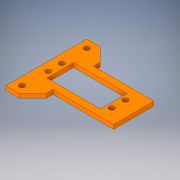
# Autodesk Inventor part: Pinza_sostenedor
Saved by Autodesk Inventor 2019 (Build 230136000, 136)
## iProperties
Created: 2020-02-07
Part Number: Pinza_sostenedor
Material: Generic
Document SubType Name: Modeling
Designer: Omar
Density: 1 g/cm^3
Appearance: Default
Author: Omar
Autodesk Inventor part; units mm, degrees
ref_plane "YZ Plane" through (0, 0, 0) normal (1, 0, 0) x (0, 1, 0)
ref_plane "XZ Plane" through (0, 0, 0) normal (0, 1, 0) x (-1, 0, 0)
ref_plane "XY Plane" through (0, 0, 0) normal (0, 0, 1) x (1, 0, 0)
sketch "Sketch2" plane through (0, 0, 0) normal (0, 1, 0) x (-1, 0, 0)
  circle A0 centre (-33.79, -5.085) radius 2
  circle A1 centre (-33.79, 5.085) radius 2
  circle A2 centre (13.47, -5.085) radius 2
  circle A3 centre (13.47, 5.085) radius 2
  line L0 (20, 15) -> (-45, 15)
  line L1 (-45, 15) -> (-45, -15)
  line L2 (-45, -15) -> (20, -15)
  line L3 (20, -15) -> (20, 15)
  line L4 (20, 30) -> (0, 30)
  line L5 (0, -30) -> (20, -30)
  line L6 (20, -30) -> (20, 30)
  circle A4 centre (14, 24) radius 2
  circle A5 centre (14, -24) radius 2
  line L7 (0, 30) -> (0, 15)
  line L8 (0, -30) -> (0, -15)
  line L9 (9.66, 9.91) -> (-30.22, 9.91)
  line L10 (-30.22, 9.91) -> (-30.22, -9.91)
  line L11 (-30.22, -9.91) -> (9.66, -9.91)
  line L12 (9.66, -9.91) -> (9.66, 9.91)
  point P0 (0, 0)
  dimension "d27" = 4
  dimension "d28" = 4
  dimension "d29" = 4
  dimension "d30" = 4
  dimension "d31" = 13.47
  dimension "d32" = 5.085
  dimension "d33" = 10.17
  dimension "d34" = 13.47
  dimension "d35" = 33.79
  dimension "d36" = 5.085
  dimension "d37" = 10.17
  dimension "d38" = 33.79
  dimension "d39" = 30
  dimension "d40" = 65
  dimension "d41" = 20
  dimension "d42" = 15
  dimension "d43" = 60
  dimension "d44" = 30
  dimension "d45" = 20
  dimension "d46" = 4
  dimension "d47" = 4
  dimension "d48" = 6
  dimension "d49" = 6
  dimension "d50" = 6
  dimension "d51" = 6
  dimension "d52" = 9.66
  dimension "d53" = 19.82
  dimension "d54" = 9.91
  dimension "d55" = 39.88
  constraints: 26 end point, 6 centre point, 5 parallel, 3 horizontal, 3 point on line, 2 collinear, 2 perpendicular, 1 vertical
  measures "d27" diameter of A0
  measures "d28" diameter of A1
  measures "d29" diameter of A2
  measures "d30" diameter of A3
  measures "d31" horizontal distance of A2.centre point (0, 0)
  measures "d32" vertical distance of A2.centre point (0, 0)
  measures "d33" distance of A3.centre A2.centre
  measures "d34" horizontal distance of point (0, 0) A3.centre
  measures "d35" horizontal distance of A1.centre point (0, 0)
  measures "d36" vertical distance of A1.centre point (0, 0)
  measures "d37" distance of A0.centre A1.centre
  measures "d38" horizontal distance of point (0, 0) A0.centre
  measures "d39" distance of L0.end L1.end
  measures "d40" distance of L0.start L0.end
  measures "d41" distance from line of L3 point (0, 0)
  measures "d42" distance from line of L0 point (0, 0)
  measures "d43" distance of L5.end L4.start
  measures "d44" distance from line of L5 point (0, 0)
  measures "d45" distance of L5.start L5.end
  measures "d46" diameter of A4
  measures "d47" diameter of A5
  measures "d48" distance from line of L6 A5.centre
  measures "d49" distance from line of L5 A5.centre
  measures "d50" distance from line of L6 A4.centre
  measures "d51" distance from line of L4 A4.centre
  measures "d52" distance from line of L12 point (0, 0)
  measures "d53" distance of L11.end L9.start
  measures "d54" distance from line of point (0, 0) L11
  measures "d55" distance of L10.end L11.end
extrude "Extrusion2" add sketch "Sketch2" along normal blind 3.18
chamfer "Chamfer1" distance 10 angle 45 1 edges at (0, 1.59, -30)
chamfer "Chamfer2" distance 10 angle 45 1 edges at (0, 1.59, 30)
body "Solid2"
